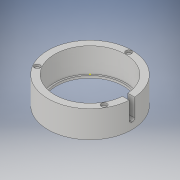
# Autodesk Inventor part: Sensor63Deckel
Saved by Autodesk Inventor 2017 (Build 210142000, 142)
## iProperties
Part Number: Sensor63Deckel
Material: Generisch
Document SubType Name: Modeling
Designer: Harald.Noeske
Density: 1 g/cm^3
Appearance: Vorgabe
Author: Harald.Noeske
Autodesk Inventor part; units mm, degrees
ref_plane "YZ Plane" through (0, 0, 0) normal (1, 0, 0) x (0, 1, 0)
ref_plane "XZ Plane" through (0, 0, 0) normal (0, 1, 0) x (-1, 0, 0)
ref_plane "XY Plane" through (0, 0, 0) normal (0, 0, 1) x (1, 0, 0)
sketch "Skizze1" plane through (0, 0, 0) normal (0, 0, 1) x (1, 0, 0)
  circle A0 centre (0, 0) radius 31.5
  circle A1 centre (0, 0) radius 37.5
  dimension "d0" = 63
  dimension "d1" = 75
  constraints: 2 centre point, 2 coincident
  measures "d0" diameter of A0
  measures "d1" diameter of A1
extrude "Extrusion1" add sketch "Skizze1" along normal blind 22
sketch "Skizze2" plane through (0, 0, 0) normal (0, 0, -1) x (-1, 0, 0)
  circle A0 centre (0, 0) radius 37.5
  circle A1 centre (0, 0) radius 30
  dimension "d4" = 75
  dimension "d5" = 60
  constraints: 2 centre point, 2 coincident
  measures "d4" diameter of A0
  measures "d5" diameter of A1
extrude "Extrusion2" add sketch "Skizze2" along normal blind 2
sketch "Skizze3" plane through (0, 0, 22) normal (0, 0, 1) x (1, 0, 0)
  point P0 (0, 0)
  point P1 (0, 34.5)
  dimension "d8" = 34.5
  measures "d8" distance of point (0, 34.5) point (0, 0)
hole "Bohrung1" at (0, 34.5, 22) direction (0, 0, -1) diameter 5.05 depth 2.1
pattern_circular "Runde Anordnung1" count 3 over 360 about axis through (0, 0, 0) along (0, 0, 1) of "Bohrung1"
sketch "Skizze4" plane through (0, 0, 22) normal (0, 0, 1) x (1, 0, 0)
  line L0 (14.3077, 2.4) -> (40, 2.4)
  line L1 (40, 2.4) -> (40, -2.4)
  line L2 (40, -2.4) -> (14.3077, -2.4)
  line L3 (14.3077, -2.4) -> (14.3077, 2.4)
  point P0 (0, 0)
  dimension "d19" = 4.8
  dimension "d20" = 2.4
  dimension "d21" = 40
  constraints: 8 end point, 2 parallel, 1 horizontal, 1 perpendicular
  measures "d19" distance of L0.end L1.end
  measures "d20" distance from line of L2 point (0, 0)
  measures "d21" horizontal distance of L1.end point (0, 0)
extrude "Extrusion3" cut sketch "Skizze4" against normal blind 18
fillet "Rundung1" radius 2 2 edges at (34.4158, 2.4, 4) (34.4158, -2.4, 4)
sketch "Skizze5" plane through (0, 0, 22) normal (0, 0, 1) x (1, 0, 0)
  point P0 (0, 0)
equation "\"d20\" = 0.5 * d19"
